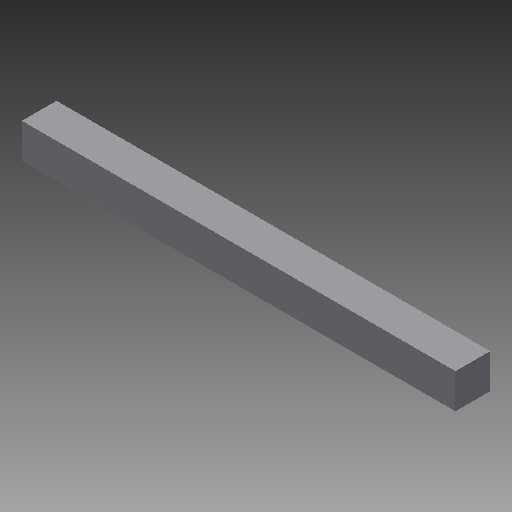
# Autodesk Inventor part: Stick
Saved by Autodesk Inventor 2018 (Build 220112000, 112)
## iProperties
Created: 2018-12-21
Part Number: Stick
Material: Типовые
Document SubType Name: Modeling
Designer: kostya
Density: 1 g/cm^3
Appearance: По умолчанию
Author: kostya
Autodesk Inventor part; units mm, degrees
ref_plane "YZ Plane" through (0, 0, 0) normal (1, 0, 0) x (0, 1, 0)
ref_plane "XZ Plane" through (0, 0, 0) normal (0, 1, 0) x (-1, 0, 0)
ref_plane "XY Plane" through (0, 0, 0) normal (0, 0, 1) x (1, 0, 0)
sketch "Эскиз1" plane through (0, 0, 0) normal (1, 0, 0) x (0, 1, 0)
  line L0 (-10, -10) -> (10, -10)
  line L1 (10, -10) -> (10, 10)
  line L2 (10, 10) -> (-10, 10)
  line L3 (-10, 10) -> (-10, -10)
  line L4 (-10, -10) -> (10, 10) construction
  line L5 (10, -10) -> (-10, 10) construction
  point P0 (0, 0)
  dimension "d0" = 20
  dimension "d1" = 20
  constraints: 12 end point, 2 midpoint, 2 parallel, 1 horizontal, 1 perpendicular
  measures "d0" distance of L2.end L1.end
  measures "d1" distance of L1.end L0.end
extrude "Выдавливание1" add sketch "Эскиз1" along normal blind 250
sketch "Эскиз2" plane through (250, 0, 0) normal (1, 0, 0) x (0, 0, -1)
  line L0 (-10, -10) -> (-10, 10)
  point P0 (0, 0)
  constraints: 2 end point, 1 vertical
sketch "Эскиз3" plane through (0, -10, -10) normal (0, -1, 0) x (1, 0, 0)
  line L0 (0, 20) -> (0, 0) projected
  line L1 (0, 0) -> (250, 0) projected
  line L2 (250, 20) -> (250, 0) projected
  line L3 (0, 20) -> (250, 20) projected
  line L4 (0, 0) -> (0, -100) construction
  line L5 (250, 0) -> (250, -100) construction
  point P0 (0, 10)
  dimension "d4" = 100
  dimension "d6" = 100
  constraints: 4 end point, 2 vertical
  measures "d4" distance of L0.end L4.end
  measures "d6" distance of L1.end L5.end
sketch "Эскиз4" plane through (0, 10, 10) normal (0, 1, 0) x (1, 0, 0)
  line L0 (0, 19.9024) -> (0, 119.9024) construction
  point P0 (0, 10)
  dimension "d7" = 100
  constraints: 2 end point, 1 vertical
  measures "d7" distance of L0.start L0.end
sketch3d "3D эскиз1"
ref_plane "РабПлоскость1" through (0, -10, -110) normal (0, 0.0048779, -0.9999881) x (0, 0.9999881, 0.0048779)
